Autodesk Inventor part; units mm, degrees
(part 2 of 2)
  spline S182 degree 2 poles (4.0705, 37.4541) (4.5938, 37.4541) (5.3962, 38.2515) (5.3962, 38.8246) knots 0 0 0 1 2 2 2
  spline S183 degree 2 poles (5.3962, 38.8246) (5.3962, 39.3778) (4.6835, 40.3397) (4.0556, 40.5988) knots 0 0 0 1 2 2 2
  spline S184 degree 2 poles (4.0556, 40.5988) (3.5672, 40.8031) (2.72, 40.833) knots 0 0 0 1 1 1
  line L105 (2.72, 40.833) -> (3.8911, 43.2003)
  line L106 (3.8911, 43.2003) -> (6.0789, 43.2003)
  point P0 (0, 0)
  constraints: 2 other
extrude "Extrusion16" add sketch "Sketch15" along normal blind 3
body "Solid1"
